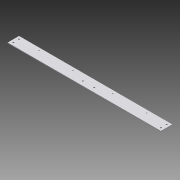
# Autodesk Inventor part: 2x2 angle rail support
Saved by Autodesk Inventor 2015 (Build 190159000, 159)
## iProperties
Created: 2015-01-27
Part Number: 2x2 angle rail support
Material: Aluminum 6061
Document SubType Name: Modeling
Designer: Admin
Density: 2.7 g/cm^3
Appearance: Aluminum - Flat
Author: Admin
Autodesk Inventor part; units mm, degrees
ref_plane "YZ Plane" through (0, 0, 0) normal (1, 0, 0) x (0, 1, 0)
ref_plane "XZ Plane" through (0, 0, 0) normal (0, 1, 0) x (-1, 0, 0)
ref_plane "XY Plane" through (0, 0, 0) normal (0, 0, 1) x (1, 0, 0)
sketch "Sketch1" plane through (0, 0, 0) normal (1, 0, 0) x (0, 1, 0)
  line L0 (0, 0) -> (-3.175, 0)
  line L1 (-3.175, 0) -> (-3.175, 50.8)
  line L2 (-3.175, 50.8) -> (0, 50.8)
  line L3 (0, 50.8) -> (0, 0)
  line L4 (0, 0) -> (-50.8, 0)
  line L5 (-50.8, 0) -> (-50.8, 3.175)
  line L6 (-50.8, 3.175) -> (0, 3.175)
  line L7 (0, 3.175) -> (0, 0)
  dimension "d0" = 3.175
  dimension "d1" = 50.8
  dimension "d2" = 50.8
  dimension "d3" = 3.175
  constraints: 16 end point, 4 parallel, 2 horizontal, 2 perpendicular
  measures "d0" distance of L1.end L2.end
  measures "d1" distance of L0.end L1.end
  measures "d2" distance of L5.end L6.end
  measures "d3" distance of L4.end L5.end
extrude "Extrusion1" add sketch "Sketch1" along normal blind 685.8
sketch "Sketch2" plane through (0, -50.8, 3.175) normal (0, 0, 1) x (1, 0, 0)
  line L0 (0, 47.625) -> (0, 0) projected
  line L1 (0, 0) -> (685.8, 0) projected
  point P0 (0, 50.8)
  point P1 (206.375, 12.7)
  point P2 (479.425, 12.7)
  point P3 (219.075, 12.7)
  point P4 (466.725, 12.7)
  dimension "d9" = 12.7
  dimension "d11" = 12.7
  dimension "d117" = 12.7
  dimension "d118" = 12.7
  dimension "d121" = 12.7
  dimension "d122" = 12.7
  dimension "d130" = 206.375
  dimension "d131" = 247.65
  measures "d9" distance from line of L1 point (206.375, 12.7)
  measures "d11" distance from line of L1 point (479.425, 12.7)
  measures "d117" distance of point (206.375, 12.7) point (219.075, 12.7)
  measures "d118" distance from line of L1 point (219.075, 12.7)
  measures "d121" distance of point (479.425, 12.7) point (466.725, 12.7)
  measures "d122" distance from line of L1 point (466.725, 12.7)
  measures "d130" distance from line of L0 point (206.375, 12.7)
  measures "d131" distance of point (219.075, 12.7) point (466.725, 12.7)
sketch "Sketch3" plane through (0, 0, 50.8) normal (0, 1, 0) x (1, 0, 0)
  line L0 (0, 50.8) -> (0, 0) projected
  line L1 (0, 0) -> (685.8, 0) projected
  line L2 (685.8, 50.8) -> (685.8, 0) projected
  line L3 (0, 50.8) -> (685.8, 50.8) projected
  point P0 (12.7, 12.7)
  point P1 (12.7, 38.1)
  point P2 (317.5, 19.05)
  point P3 (368.3, 19.05)
  point P4 (673.1, 12.7)
  point P5 (673.1, 38.1)
  dimension "d19" = 12.7
  dimension "d20" = 12.7
  dimension "d21" = 12.7
  dimension "d22" = 12.7
  dimension "d23" = 19.05
  dimension "d24" = 19.05
  dimension "d25" = 12.7
  dimension "d26" = 12.7
  dimension "d27" = 12.7
  dimension "d28" = 12.7
  dimension "d29" = 317.5
  dimension "d30" = 317.5
  measures "d19" distance from line of L1 point (12.7, 12.7)
  measures "d20" distance from line of L0 point (12.7, 12.7)
  measures "d21" distance from line of L0 point (12.7, 38.1)
  measures "d22" distance from line of L3 point (12.7, 38.1)
  measures "d23" distance from line of L1 point (317.5, 19.05)
  measures "d24" distance from line of L1 point (368.3, 19.05)
  measures "d25" distance from line of L1 point (673.1, 12.7)
  measures "d26" distance from line of L2 point (673.1, 12.7)
  measures "d27" distance from line of L2 point (673.1, 38.1)
  measures "d28" distance from line of L3 point (673.1, 38.1)
  measures "d29" distance from line of L2 point (368.3, 19.05)
  measures "d30" distance from line of L0 point (317.5, 19.05)
hole "Hole2" at (12.7, 0, 38.1) at (12.7, 0, 12.7) at (317.5, 0, 31.75) at (368.3, 0, 31.75) at (673.1, 0, 38.1) at (673.1, 0, 12.7) direction (0, -1, 0) diameter 6.35 end through all
sketch "Sketch4" plane through (0, 0, 50.8) normal (0, 1, 0) x (1, 0, 0)
  line L0 (0, 50.8) -> (0, 0) projected
  line L1 (685.8, 50.8) -> (685.8, 0) projected
  line L2 (0, 50.8) -> (685.8, 50.8) projected
  point P0 (101.6, 38.1)
  point P1 (254, 38.1)
  point P2 (431.8, 38.1)
  point P3 (584.2, 38.1)
  dimension "d38" = 101.6
  dimension "d39" = 254
  dimension "d40" = 254
  dimension "d41" = 101.6
  dimension "d42" = 12.7
  dimension "d43" = 12.7
  dimension "d44" = 12.7
  dimension "d45" = 12.7
  measures "d38" distance from line of L0 point (101.6, 38.1)
  measures "d39" distance from line of L0 point (254, 38.1)
  measures "d40" distance from line of L1 point (431.8, 38.1)
  measures "d41" distance from line of L1 point (584.2, 38.1)
  measures "d42" distance from line of L2 point (431.8, 38.1)
  measures "d43" distance from line of L2 point (584.2, 38.1)
  measures "d44" distance from line of L2 point (254, 38.1)
  measures "d45" distance from line of L2 point (101.6, 38.1)
hole "Hole3" at (101.6, 0, 12.7) at (254, 0, 12.7) at (431.8, 0, 12.7) at (584.2, 0, 12.7) direction (0, -1, 0) diameter 4.7625 end through all
sketch "Sketch6" plane through (0, -50.8, 0) normal (0, 0, -1) x (-1, 0, 0)
  line L0 (0, 0) -> (0, 50.8) projected
  line L1 (-685.8, 0) -> (-685.8, 50.8) projected
  line L2 (-685.8, 0) -> (-533.4, 0)
  line L3 (-533.4, 0) -> (-533.4, 25.4)
  line L4 (-533.4, 25.4) -> (-685.8, 25.4)
  line L5 (-685.8, 25.4) -> (-685.8, 0)
  line L6 (0, 0) -> (-152.4, 0)
  line L7 (-152.4, 0) -> (-152.4, 25.4)
  line L8 (-152.4, 25.4) -> (0, 25.4)
  line L9 (0, 25.4) -> (0, 0)
  line L10 (-685.8, 47.625) -> (-663.575, 25.4)
  line L11 (-685.8, 47.625) -> (-654.3691, 47.625) construction
  line L12 (-663.575, 25.4) -> (-685.8, 25.4)
  line L13 (-685.8, 25.4) -> (-685.8, 47.625)
  line L14 (0, 47.625) -> (-22.225, 25.4)
  line L15 (0, 47.625) -> (31.4309, 47.625) construction
  line L16 (-22.225, 25.4) -> (0, 25.4)
  line L17 (0, 25.4) -> (0, 47.625)
  line L18 (0, 47.625) -> (-685.8, 47.625) projected
  dimension "d65" = 152.4
  dimension "d66" = 25.4
  dimension "d67" = 152.4
  dimension "d68" = 25.4
  dimension "d69" = 45
  dimension "d70" = 135
  constraints: 32 end point, 6 perpendicular, 4 horizontal, 4 parallel, 2 equal length, 2 point on line
  measures "d65" distance of L4.end L3.end
  measures "d66" distance of L3.end L2.end
  measures "d67" distance of L7.end L8.end
  measures "d68" distance of L6.end L7.end
  measures "d69" angle of L10 L11
  measures "d70" angle of L14 L15
extrude "Extrusion3" cut sketch "Sketch6" against normal blind 25.4
chamfer "Chamfer1" distance 3.175 angle 45 2 edges at (533.4, -50.8, 1.5875) (152.4, -50.8, 1.5875)
sketch "Sketch8" plane through (685.8, 0, 0) normal (0, 0, -1) x (-1, 0, 0)
  line L0 (685.8, 0) -> (0, 0) projected
  line L1 (0, -3.175) -> (0, 0) projected
  point P0 (101.6, -12.7)
  point P1 (254, -12.7)
  point P2 (431.8, -12.7)
  point P3 (584.2, -12.7)
  dimension "d91" = 12.7
  dimension "d92" = 12.7
  dimension "d93" = 12.7
  dimension "d94" = 12.7
  dimension "d95" = 101.6
  dimension "d96" = 254
  dimension "d97" = 431.8
  dimension "d98" = 584.2
  measures "d91" distance from line of L0 point (101.6, -12.7)
  measures "d92" distance from line of L0 point (254, -12.7)
  measures "d93" distance from line of L0 point (431.8, -12.7)
  measures "d94" distance from line of L0 point (584.2, -12.7)
  measures "d95" distance from line of L1 point (101.6, -12.7)
  measures "d96" distance from line of point (254, -12.7) L1
  measures "d97" distance from line of point (431.8, -12.7) L1
  measures "d98" distance from line of L1 point (584.2, -12.7)
hole "Hole5" at (584.2, -12.7, 0) at (431.8, -12.7, 0) at (254, -12.7, 0) at (101.6, -12.7, 0) direction (0, 0, 1) diameter 4.7625 end through all
sketch "Sketch9" plane through (0, -3.175, 3.175) normal (0, 0, 1) x (1, 0, 0)
  line L0 (0, 0) -> (685.8, 0) projected
  line L1 (0, 3.175) -> (0, 0) projected
  line L2 (685.8, 0) -> (685.8, 3.175) projected
  point P0 (203.2, -6.35)
  point P1 (482.6, -6.35)
  dimension "d106" = 203.2
  dimension "d107" = 6.35
  dimension "d108" = 6.35
  dimension "d109" = 203.2
  measures "d106" distance from line of L1 point (203.2, -6.35)
  measures "d107" distance from line of L0 point (203.2, -6.35)
  measures "d108" distance from line of L0 point (482.6, -6.35)
  measures "d109" distance from line of L2 point (482.6, -6.35)
hole "Hole6" at (203.2, -9.525, 3.175) at (482.6, -9.525, 3.175) direction (0, 0, -1) diameter 9.525 depth 25.4 tip angle 118
hole "Hole7" at (206.375, -38.1, 3.175) at (479.425, -38.1, 3.175) at (219.075, -38.1, 3.175) at (466.725, -38.1, 3.175) direction (0, 0, -1) diameter 6.35 depth 25.4 tip angle 118
body "Solid1"
